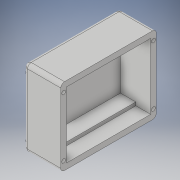
# Autodesk Inventor part: bottom
Saved by Autodesk Inventor 2017 (Build 210142000, 142)
## iProperties
Created: 2018-05-31
Part Number: bottom
Material: Generic
Document SubType Name: Modeling
Designer: sinner
Density: 1 g/cm^3
Appearance: Default
Author: sinner
Autodesk Inventor part; units mm, degrees
ref_plane "YZ Plane" through (0, 0, 0) normal (1, 0, 0) x (0, 1, 0)
ref_plane "XZ Plane" through (0, 0, 0) normal (0, 1, 0) x (-1, 0, 0)
ref_plane "XY Plane" through (0, 0, 0) normal (0, 0, 1) x (1, 0, 0)
sketch "Sketch1" plane through (0, 0, 0) normal (1, 0, 0) x (0, 1, 0)
  line L0 (0, 0) -> (66.04, 0)
  line L1 (66.04, 0) -> (66.04, -81.915)
  line L2 (66.04, -81.915) -> (0, -81.915)
  line L3 (0, -81.915) -> (0, 0)
  dimension "d0" = 66.04
  dimension "d1" = 81.915
  constraints: 8 end point, 2 parallel, 1 horizontal, 1 perpendicular
  measures "d0" distance of L1.end L2.end
  measures "d1" distance of L0.end L1.end
extrude "Extrusion1" add sketch "Sketch1" along normal blind 31.75
fillet "Fillet1" radius 3.175 4 edges at (15.875, 0, -81.915) (15.875, 66.04, -81.915) (15.875, 0, 0) (15.875, 66.04, 0)
sketch "Sketch2" plane through (31.75, 0, 0) normal (1, 0, 0) x (0, 0, -1)
  line L0 (77.1525, 4.7625) -> (4.7625, 4.7625)
  line L1 (4.7625, 4.7625) -> (4.7625, 61.2775)
  line L2 (4.7625, 61.2775) -> (77.1525, 61.2775)
  line L3 (77.1525, 61.2775) -> (77.1525, 4.7625)
  line L4 (0, 0) -> (20.3539, 0) construction
  line L5 (3.175, 0) -> (78.74, 0) projected
  line L6 (0, 0) -> (0, 12.4806) construction
  line L7 (0, 62.865) -> (0, 3.175) projected
  dimension "d6" = 56.515
  dimension "d7" = 72.39
  dimension "d10" = 4.7625
  dimension "d19" = 4.7625
  constraints: 12 end point, 2 parallel, 2 point on line, 1 horizontal, 1 perpendicular
  measures "d6" distance of L0.end L1.end
  measures "d7" distance of L0.start L0.end
  measures "d10" distance between parallel lines of L6 L1
  measures "d19" distance between parallel lines of L4 L0
extrude "Extrusion2" cut sketch "Sketch2" against normal blind 12.7
sketch "Sketch3" plane through (19.05, 0, 0) normal (1, 0, 0) x (0, 0, -1)
  line L0 (77.1525, 61.2775) -> (77.1525, 4.7625) projected
  line L1 (77.1525, 33.02) -> (4.7625, 33.02) construction
  line L2 (4.7625, 4.7625) -> (4.7625, 61.2775) projected
  line L3 (4.7625, 7.62) -> (77.1525, 7.62)
  line L4 (77.1525, 7.62) -> (77.1525, 58.42)
  line L5 (77.1525, 58.42) -> (4.7625, 58.42)
  line L6 (4.7625, 58.42) -> (4.7625, 7.62)
  line L7 (4.7625, 7.62) -> (77.1525, 58.42) construction
  line L8 (77.1525, 7.62) -> (4.7625, 58.42) construction
  line L9 (77.1525, 4.7625) -> (4.7625, 4.7625) projected
  line L10 (77.1525, 4.7625) -> (77.1525, 24.7395)
  point P0 (40.9575, 33.02)
  dimension "d11" = 50.8
  dimension "d12" = 72.39
  constraints: 16 end point, 5 midpoint, 2 parallel, 1 collinear, 1 horizontal, 1 perpendicular
  measures "d11" distance of L3.end L4.end
  measures "d12" distance of L4.end L5.end
extrude "Extrusion3" cut sketch "Sketch3" against normal blind 13.208 contours L0 L3 L2 L5
fillet "Fillet3" radius 3.175 8 edges at (0, 0.9299, -80.9851) (0, 0, -40.9575) (0, 0.9299, -0.9299) (0, 33.02, 0) (0, 65.1101, -0.9299) (0, 66.04, -40.9575) (0, 65.1101, -80.9851) (0, 33.02, -81.915)
sketch "Sketch4" plane through (31.75, 0, 0) normal (1, 0, 0) x (0, 0, -1)
  line L0 (2.3813, -0.2223) -> (2.3813, 65.5235) construction
  line L1 (0, 3.175) -> (0, 62.865) projected
  circle A0 centre (2.3813, 7.62) radius 1.632
  line L2 (0, 62.865) -> (0, 3.175) projected
  line L3 (0, 33.02) -> (4.7625, 33.02) construction
  line L4 (4.7625, 7.62) -> (4.7625, 58.42) projected
  circle A1 centre (2.3812, 58.42) radius 1.632
  line L5 (4.7625, 58.42) -> (4.7625, 7.62)
  line L6 (77.1525, 4.7625) -> (4.7625, 4.7625) projected
  line L7 (40.9575, 4.7625) -> (40.9575, -0.2223) construction
  circle A2 centre (79.5338, 7.62) radius 1.632
  circle A3 centre (79.5338, 58.42) radius 1.632
  point P0 (0, 0)
  dimension "d17" = 2.3813
  dimension "d18" = 3.2639
  dimension "d21" = 25.4
  constraints: 8 end point, 5 symmetric about line, 4 centre point, 3 midpoint, 2 vertical, 1 point on line, 3 other
  measures "d17" distance between parallel lines of L1 L0
  measures "d18" diameter of A0
  measures "d21" distance from line of L3 A0.centre
extrude "Extrusion4" cut sketch "Sketch4" against normal blind 31.75
body "Solid1"
